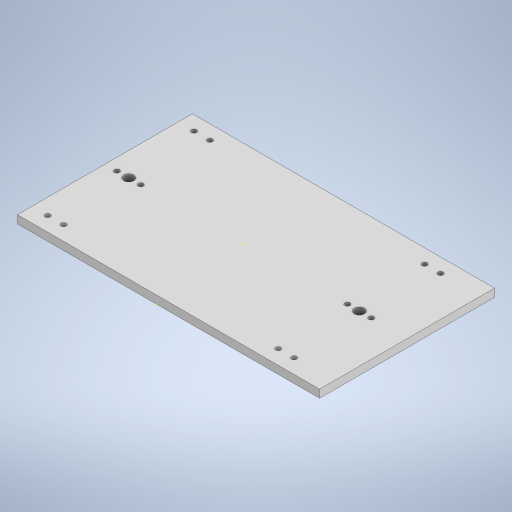
# Autodesk Inventor part: Base Plate
Saved by Autodesk Inventor 2023 (Build 270158000, 158)
## iProperties
Created: 2023-02-08
Part Number: Base Plate
Material: Generic
Document SubType Name: Modeling
Designer: deepa
Density: 1 g/cm^3
Appearance: Default
Author: deepa
Autodesk Inventor part; units mm, degrees
ref_plane "YZ Plane" through (0, 0, 0) normal (1, 0, 0) x (0, 1, 0)
ref_plane "XZ Plane" through (0, 0, 0) normal (0, 1, 0) x (-1, 0, 0)
ref_plane "XY Plane" through (0, 0, 0) normal (0, 0, 1) x (1, 0, 0)
sketch "Sketch1" plane through (0, 0, 0) normal (0, 1, 0) x (-1, 0, 0)
  point P0 (0, 0)
sketch "Sketch2" plane through (0, 0, 0) normal (0, 1, 0) x (-1, 0, 0)
  line L0 (175, 110) -> (-205, 110)
  line L1 (-205, 110) -> (-205, -110)
  line L2 (-205, -110) -> (175, -110)
  line L3 (175, -110) -> (175, 110)
  point P0 (0, 0)
  point P1 (0, 0)
  dimension "d0" = 380
  dimension "d1" = 220
  dimension "d2" = 110
  dimension "d3" = 175
  constraints: 8 end point, 2 parallel, 1 coincident, 1 horizontal, 1 perpendicular
  measures "d0" distance of L2.end L1.end
  measures "d1" distance of L1.end L0.end
  measures "d2" distance from line of L0 point (0, 0)
  measures "d3" distance from line of L3 point (0, 0)
extrude "Extrusion1" add sketch "Sketch2" along normal blind 10
sketch "Sketch3" plane through (0, 10, 0) normal (0, 1, 0) x (1, 0, 0)
  circle A0 centre (-145, 0) radius 6.35
  circle A1 centre (145, 0) radius 6.35
  line L0 (-175, 110) -> (-175, -110) projected
  circle A2 centre (-160, 0) radius 3.25
  circle A3 centre (-130, 0) radius 3.25
  circle A4 centre (160, 0) radius 3.25
  circle A5 centre (130, 0) radius 3.25
  line L1 (-145, -118.0752) -> (-145, 98.7202) construction
  circle A6 centre (-155, -92) radius 3.25
  line L2 (-145, -65.9248) -> (-145, -282.7202) construction
  circle A7 centre (-135, -92) radius 3.25
  circle A8 centre (-155, 92) radius 3.25
  circle A9 centre (-135, 92) radius 3.25
  circle A10 centre (155, 92) radius 3.25
  circle A11 centre (135, 92) radius 3.25
  circle A12 centre (155, -92) radius 3.25
  circle A13 centre (135, -92) radius 3.25
  line L3 (-175, -110) -> (205, -110) projected
  point P0 (0, 0)
  point P1 (-145, -92)
  point P2 (-145, -92)
  dimension "d6" = 12.7
  dimension "d9" = 360
  dimension "d11" = 30
  dimension "d12" = 6.5
  dimension "d15" = 360
  dimension "d19" = 360
  dimension "d21" = 15
  dimension "d22" = 6.5
  dimension "d25" = 360
  dimension "d29" = 360
  dimension "d33" = 360
  dimension "d35" = 220
  dimension "d36" = 18
  dimension "d37" = 18
  dimension "d41" = 10
  constraints: 14 centre point, 4 end point, 2 coincident, 2 point on line, 1 vertical, 56 other
  measures "d6" diameter of A0
  measures "d11" distance from line of A0.centre L0
  measures "d12" diameter of A2
  measures "d21" distance of A0.centre A2.centre
  measures "d22" diameter of A6
  measures "d35" distance of L0.start L0.end
  measures "d36" distance from line of L3 A7.centre
  measures "d37" distance from line of L3 point (-145, -92)
  measures "d41" distance from line of A6.centre L2
extrude "Extrusion2" cut sketch "Sketch3" against normal blind 10
sketch "Sketch4" plane through (-175, 0, 110) normal (0, 0, 1) x (1, 0, 0)
  point P0 (175, 0)
sketch "Sketch5" plane through (0, 10, 0) normal (0, 1, 0) x (1, 0, 0)
  point P0 (0, 0)
body "Solid1"
